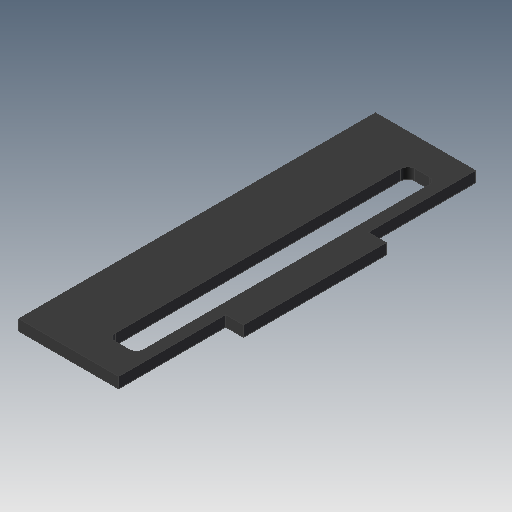
# Autodesk Inventor part: Lateral BNC
Saved by Autodesk Inventor 2020 (Build 240168000, 168)
## iProperties
Created: 2020-11-07
Part Number: Lateral BNC
Material: Generic
Document SubType Name: Modeling
Designer: ferrerx
Density: 1 g/cm^3
Appearance: Default
Author: ferrerx
Autodesk Inventor part; units mm, degrees
ref_plane "YZ Plane" through (0, 0, 0) normal (1, 0, 0) x (0, 1, 0)
ref_plane "XZ Plane" through (0, 0, 0) normal (0, 1, 0) x (-1, 0, 0)
ref_plane "XY Plane" through (0, 0, 0) normal (0, 0, 1) x (1, 0, 0)
sketch "Sketch1" plane through (0, 0, 0) normal (0, 1, 0) x (-1, 0, 0)
  line L0 (0, 0) -> (28, 0)
  line L1 (28, 0) -> (28, -100)
  line L2 (28, -100) -> (0, -100)
  line L3 (0, -100) -> (0, 0)
  line L4 (0, -30) -> (-5, -30)
  line L5 (-5, -30) -> (-5, -70)
  line L6 (-5, -70) -> (0, -70)
  line L7 (0, -70) -> (0, -30)
  line L8 (28, -50) -> (0, -50) construction
  line L9 (-5, -50) -> (0, -50) construction
  point P0 (0, -70)
  dimension "d0" = 100
  dimension "d1" = 5
  dimension "d2" = 40
  dimension "d3" = 28
  constraints: 20 end point, 4 midpoint, 4 parallel, 2 horizontal, 2 perpendicular, 1 collinear, 1 point on line
  measures "d0" distance of L2.end L0.start
  measures "d1" distance of L5.end L6.end
  measures "d2" distance of L4.end L5.end
  measures "d3" distance of L1.end L2.end
extrude "Extrusion1" add sketch "Sketch1" along normal blind 3
sketch "Sketch4" plane through (0, 3, 0) normal (0, 1, 0) x (1, 0, 0)
  line L0 (-3, 92) -> (-11, 92)
  line L1 (-11, 92) -> (-11, 8)
  line L2 (-11, 8) -> (-3, 8)
  line L3 (-3, 8) -> (-3, 92)
  line L4 (0, 70) -> (0, 100) projected
  line L5 (0, 100) -> (-28, 100) projected
  point P0 (0, 0)
  dimension "d24" = 3
  dimension "d25" = 8
  dimension "d26" = 84
  dimension "d27" = 8
  constraints: 8 end point, 2 parallel, 1 horizontal, 1 perpendicular
  measures "d24" distance between parallel lines of L4 L3
  measures "d25" distance of L0.start L0.end
  measures "d26" distance of L0.end L1.end
  measures "d27" distance between parallel lines of L5 L0
extrude "Extrusion4" cut sketch "Sketch4" against normal blind 10
fillet "Fillet1" radius 2 4 edges at (-11, 1.5, -92) (-3, 1.5, -92) (-11, 1.5, -8) (-3, 1.5, -8)
body "Solid1"
